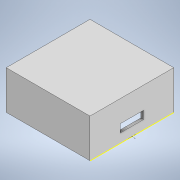
# Autodesk Inventor part: snapfit_lid_v10
Saved by Autodesk Inventor 2022 (Build 260153000, 153)
## iProperties
Created: 2022-03-20
Part Number: snapfit_lid_v10
Material: Generic
Document SubType Name: Modeling
Designer: LIMlab
Density: 1 g/cm^3
Appearance: Default
Author: LIMlab
Autodesk Inventor part; units mm, degrees
ref_plane "YZ Plane" through (0, 0, 0) normal (1, 0, 0) x (0, 1, 0)
ref_plane "XZ Plane" through (0, 0, 0) normal (0, 1, 0) x (-1, 0, 0)
ref_plane "XY Plane" through (0, 0, 0) normal (0, 0, 1) x (1, 0, 0)
sketch "Sketch2" plane through (0, 0, 0) normal (0, 1, 0) x (-1, 0, 0)
  line L0 (-2.75, -2.75) -> (2.75, -2.75)
  line L1 (2.75, -2.75) -> (2.75, 2.75)
  line L2 (2.75, 2.75) -> (-2.75, 2.75)
  line L3 (-2.75, 2.75) -> (-2.75, -2.75)
  line L4 (-2.75, -2.75) -> (2.75, 2.75) construction
  line L5 (2.75, -2.75) -> (-2.75, 2.75) construction
  line L6 (3.25, 3.25) -> (-3.25, 3.25)
  line L7 (-3.25, 3.25) -> (-3.25, -3.25)
  line L8 (-3.25, -3.25) -> (3.25, -3.25)
  line L9 (3.25, -3.25) -> (3.25, 3.25)
  line L10 (3.25, 3.25) -> (-3.25, -3.25) construction
  line L11 (-3.25, 3.25) -> (3.25, -3.25) construction
  point P0 (0, 0)
  point P1 (3.25, 0)
  point P2 (-3.25, 0)
  point P3 (3.25, 0)
  point P4 (-3.25, 0)
  point P5 (3.25, 0)
  point P6 (2.75, 0)
  point P7 (-2.75, 0)
  dimension "d2" = 5.5
  dimension "d3" = 5.5
  dimension "d6" = 6.5
  dimension "d7" = 6.5
  constraints: 24 end point, 8 midpoint, 4 parallel, 3 coincident, 2 horizontal, 2 perpendicular
  measures "d2" distance of L2.end L1.end
  measures "d3" distance of L1.end L0.end
  measures "d6" distance of L8.end L7.end
  measures "d7" distance of L7.end L6.end
extrude "Extrusion1" add sketch "Sketch2" along normal blind 2
sketch "Sketch4" plane through (0, 2, 0) normal (0, 1, 0) x (1, 0, 0)
  line L0 (-3.25, 3.25) -> (-3.25, -3.25) projected
  line L1 (3.25, -3.25) -> (3.25, 3.25) projected
  line L2 (-3.25, -3.25) -> (3.25, -3.25)
  line L3 (3.25, -3.25) -> (3.25, 3.25)
  line L4 (3.25, 3.25) -> (-3.25, 3.25)
  line L5 (-3.25, 3.25) -> (-3.25, -3.25)
  point P0 (0, 0)
  dimension "d10" = 6.5
  constraints: 8 end point, 2 parallel, 1 horizontal, 1 perpendicular
  measures "d10" distance of L4.end L1.end
extrude "Extrusion2" add sketch "Sketch4" along normal blind 1
sketch "Sketch5" plane through (0, 0, 0) normal (0, -1, 0) x (1, 0, 0)
  line L0 (-3.25, -3.25) -> (-3.25, 3.25) projected
  line L1 (3.25, 3.25) -> (3.25, -3.25) projected
  point P0 (0, 0)
  point P1 (-3.25, 0)
  point P2 (3.25, 0)
  constraints: 2 midpoint
sketch "Sketch6" plane through (2.75, 0, -2.75) normal (-1, 0, 0) x (0, 0, 1)
  line L0 (1.55, 0.4) -> (3.95, 0.4)
  line L1 (3.95, 0.4) -> (3.95, 1.6)
  line L2 (3.95, 1.6) -> (1.55, 1.6)
  line L3 (1.55, 1.6) -> (1.55, 0.4)
  line L4 (1.55, 0.4) -> (3.95, 1.6) construction
  line L5 (3.95, 0.4) -> (1.55, 1.6) construction
  line L6 (0, 2) -> (5.5, 2) projected
  point P0 (2.75, 0)
  point P1 (2.75, 1)
  dimension "d13" = 2.4
  dimension "d14" = 1.2
  dimension "d15" = 1
  constraints: 12 end point, 2 midpoint, 2 parallel, 1 horizontal, 1 perpendicular
  measures "d13" distance of L2.end L1.end
  measures "d14" distance of L1.end L0.end
  measures "d15" distance from line of point (2.75, 1) L6
extrude "Extrusion3" cut sketch "Sketch6" against normal blind 0.5 draft -30
sketch "Sketch7" plane through (-2.75, 0, 2.75) normal (1, 0, 0) x (0, 0, -1)
  line L0 (1.55, 0.4) -> (3.95, 0.4)
  line L1 (3.95, 0.4) -> (3.95, 1.6)
  line L2 (3.95, 1.6) -> (1.55, 1.6)
  line L3 (1.55, 1.6) -> (1.55, 0.4)
  line L4 (1.55, 0.4) -> (3.95, 1.6) construction
  line L5 (3.95, 0.4) -> (1.55, 1.6) construction
  line L6 (0, 2) -> (5.5, 2) projected
  point P0 (2.75, 0)
  point P1 (2.75, 1)
  dimension "d18" = 2.4
  dimension "d19" = 1.2
  dimension "d20" = 1
  constraints: 12 end point, 2 midpoint, 2 parallel, 1 horizontal, 1 perpendicular
  measures "d18" distance of L2.end L1.end
  measures "d19" distance of L1.end L0.end
  measures "d20" distance from line of point (2.75, 1) L6
extrude "Extrusion4" cut sketch "Sketch7" against normal blind 0.5 draft -30
body "Solid1"
